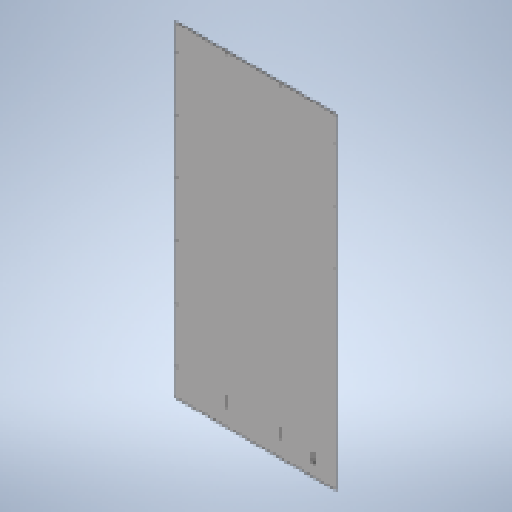
# Autodesk Inventor part: GBK 2321 shield 8
Saved by Autodesk Inventor 2026 (Build 300175000, 175)
## iProperties
Created: 2026-04-17
Part Number: GBK 2321 shield 8
Material: Steel
Document SubType Name: Sheet Metal
Designer: pokla
Stock Number: 2328
Mass: 138487 g
Surface Area: 88564.8 cm^2
Volume: 17641.6 cm^3
Density: 7.85 g/cm^3
Flat Pattern Width: 148 cm
Flat Pattern Length: 298 cm
Flat Pattern Area: 44104 cm^2
Sheet Metal Rule: По умолчанию_мм
Sheet Metal Width: 1480,000 мм
Sheet Metal Length: 2980,000 мм
Sheet Metal Area: 4410400,000 мм^2
Appearance: Default
Author: admin
Autodesk Inventor part; units mm, degrees
ref_plane "YZ Plane" through (0, 0, 0) normal (1, 0, 0) x (0, 1, 0)
ref_plane "XZ Plane" through (0, 0, 0) normal (0, 1, 0) x (-1, 0, 0)
ref_plane "XY Plane" through (0, 0, 0) normal (0, 0, 1) x (1, 0, 0)
sketch "Sketch1" plane through (0, 0, 0) normal (0, 0, 1) x (1, 0, 0)
  line L0 (740, -1490) -> (-740, -1490)
  line L1 (-740, -1490) -> (-740, 1490)
  line L2 (-740, 1490) -> (740, 1490)
  line L3 (740, 1490) -> (740, -1490)
  line L4 (740, -1490) -> (-740, 1490) construction
  line L5 (-740, -1490) -> (740, 1490) construction
  point P0 (0, 0)
  dimension "d0" = 1480
  dimension "d1" = 2980
  measures "d0" distance of L1.end L2.end
  measures "d1" distance of L0.end L1.end
extrude "Plate1" add sketch "Sketch1" along normal blind 4
sketch "Эскиз2" plane through (0, 0, 4) normal (0, 0, 1) x (1, 0, 0)
  line L0 (544.4253, -1295.3771) -> (544.4253, -1793.5133) construction
  line L1 (544.4253, -1793.5133) -> (504.798, -1793.5133) construction
  line L2 (504.798, -1793.5133) -> (504.798, -1295.3771) construction
  line L3 (504.798, -1295.3771) -> (544.4253, -1295.3771) construction
  line L4 (710, -1236) -> (710, -1232) projected
  line L5 (710, -739.3333) -> (710, -735.3333) projected
  line L6 (710, -242.6667) -> (710, -238.6667) projected
  line L7 (710, 254) -> (710, 258) projected
  line L8 (710, 750.6667) -> (710, 754.6667) projected
  line L9 (710, 1247.3333) -> (710, 1251.3333) projected
  line L10 (230.5109, -1239.5) -> (230.5109, -1336.5) projected
  line L11 (230.5109, -1336.5) -> (226.5119, -1336.5) projected
  line L12 (-269.6177, -1239.5) -> (-269.6177, -1336.5) projected
  line L13 (-269.6177, -1336.5) -> (-273.6167, -1336.5) projected
  line L14 (-739.3197, -1236) -> (-710, -1236) projected
  line L15 (-710, -1236) -> (-710, -1232) projected
  line L16 (-739.3197, -739.3333) -> (-710, -739.3333) projected
  line L17 (-710, -739.3333) -> (-710, -735.3333) projected
  line L18 (-739.3197, -242.6667) -> (-710, -242.6667) projected
  line L19 (-710, -242.6667) -> (-710, -238.6667) projected
  line L20 (-739.3197, 254) -> (-710, 254) projected
  line L21 (-710, 254) -> (-710, 258) projected
  line L22 (-739.3197, 750.6667) -> (-710, 750.6667) projected
  line L23 (-710, 750.6667) -> (-710, 754.6667) projected
  line L24 (-739.3197, 1247.3333) -> (-710, 1247.3333) projected
  line L25 (-710, 1247.3333) -> (-710, 1251.3333) projected
  ellipse E0 centre (-269.6177, 1488.5) end of major axis (-269.6177, 1518.5) minor radius 0.6803 (-269.6177, 1458.5) -> (-269.6177, 1518.5) ccw projected
  line L26 (-269.6177, 1458.5) -> (-273.6167, 1458.5) projected
  ellipse E1 centre (230.5109, 1488.5) end of major axis (230.5109, 1518.5) minor radius 0.6803 (230.5109, 1458.5) -> (230.5109, 1518.5) ccw projected
  line L27 (230.5109, 1458.5) -> (226.5119, 1458.5) projected
  point P0 (0, 0)
  constraints: 4 other
mark "Маркировка1"
equation "\"d0\" = Лист_ширина"
equation "\"d2\" = Thickness"
equation "\"BendRadius\" = Thickness"
equation "\"BendReliefWidth\" = Thickness"
equation "\"BendReliefDepth\" = 0.5 * Thickness"
equation "\"CornerReliefSize\" = 4 * Thickness"
equation "\"MinimumRemnant\" = 2 * Thickness"
equation "\"TransitionRadius\" = BendRadius"
equation "\"JacobiRadiusSize\" = BendRadius"
equation "\"GapSize\" = Thickness"
equation "\"Лист_ширина\" = 1480"
equation "\"Thickness\" = 4"
body "Solid1"
